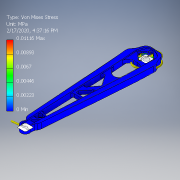
# Autodesk Inventor part: Delta_Arm
Saved by Autodesk Inventor 2019.4 (Build 234330000, 330)
## iProperties
Created: 2019-07-06
Part Number: Delta_Arm
Material: ABS Plastic
Document SubType Name: Modeling
Designer: Jorian Brusind
Density: 1.06 g/cm^3
Appearance: Chrome - Polished
Mass: 68.9986 g
Surface Area: 245.619 cm^2
Volume: 65.093 cm^3
Author: Jorian Brusind
Autodesk Inventor part; units mm, degrees
ref_plane "YZ Plane" through (0, 0, 0) normal (1, 0, 0) x (0, 1, 0)
ref_plane "XZ Plane" through (0, 0, 0) normal (0, 1, 0) x (-1, 0, 0)
ref_plane "Work Plane6" through (0, 10, 0) normal (0, 1, 0) x (1, 0, 0)
sketch "Sketch1" plane through (0, 0, 0) normal (0, 1, 0) x (-1, 0, 0)
  circle A0 centre (0, 0) radius 10
  circle A1 centre (0, -210) radius 25
  line L0 (0, -210) -> (0, 0)
  line L1 (0, 0) -> (10, 0)
  line L2 (0, 0) -> (-10, 0)
  line L3 (0, -210) -> (25, -210)
  line L4 (0, -210) -> (-25, -210)
  line L5 (25, -210) -> (10, 0)
  line L6 (-25, -210) -> (-10, 0)
  point P0 (9.9887, 0.4754)
  dimension "d0" = 20
  dimension "d2" = 50
  dimension "d50" = 210
  dimension "d51" = 210
  constraints: 14 end point, 5 point on circle, 2 centre point, 2 horizontal, 1 coincident, 1 parallel, 1 vertical
  measures "d0" diameter of A0
  measures "d2" diameter of A1
  measures "d50" distance of L0.start point (0, 0)
  measures "d51" vertical distance of L4.end L2.end
ref_plane "Work Plane5" through (0, 10, 0) normal (0, 1, 0) x (1, 0, 0)
ref_plane "Work Plane7" through (0, 10, 0) normal (0, 1, 0) x (1, 0, 0)
ref_plane "Work Plane4" through (0, 0, 0) normal (0, -1, 0) x (1, 0, 0)
ref_plane "Work Plane1" through (0, 5, 0) normal (0, -1, 0) x (1, 0, 0)
ref_plane "Work Plane3" through (0, 10, 0) normal (0, 1, 0) x (1, 0, 0)
ref_plane "Work Plane2" through (0, 0, 5) normal (0, 0, 1) x (1, 0, 0)
extrude "Extrusion8" add sketch "Sketch1" along normal blind 10 contours L1 L2 A0 | L5 A1 L0 A0 | A0 L0 L1 | L2 L0 A0 | A0 L0 A1 L6 | L5 L3 L0 A1 | A1 L0 L4 L6 | A1 L4 L3
sketch "Sketch10" plane through (0, 10, 0) normal (0, 1, 0) x (1, 0, 0)
  circle A0 centre (0, 0) radius 2
  arc A1 (25, 210) -> (-25, 210) centre (0, 210) ccw projected
  circle A2 centre (0, 210) radius 3
  dimension "d54" = 4
  dimension "d55" = 6
  constraints: 2 centre point, 2 coincident
  measures "d54" diameter of A0
  measures "d55" diameter of A2
extrude "Extrusion9" cut sketch "Sketch10" against normal blind 10
sketch "Sketch13" plane through (0, 10, 0) normal (0, 1, 0) x (1, 0, 0)
  arc A0 (-8.9826, 205.2525) -> (-4.6035, 200.9428) centre (0, 210) ccw
  arc A1 (-8.9826, 205.2525) -> (-10.7359, 206.6884) centre (-11.5651, 203.8876) ccw
  arc A2 (-10.7874, 213.1397) -> (-10.7359, 206.6884) centre (-9.7787, 209.9219) ccw
  arc A3 (-3.1397, 199.2126) -> (-4.6035, 200.9428) centre (-5.927, 198.3388) ccw
  arc A4 (-3.1397, 199.2126) -> (3.3116, 199.2641) centre (0.0781, 200.2213) ccw
  arc A5 (4.7475, 201.0174) -> (9.0572, 205.3965) centre (0, 210) ccw
  arc A6 (4.7475, 201.0174) -> (3.3116, 199.2641) centre (6.1124, 198.4349) ccw
  arc A7 (10.7874, 206.8603) -> (10.7359, 213.3116) centre (9.7787, 210.0781) ccw
  arc A8 (8.9826, 214.7475) -> (10.7359, 213.3116) centre (11.5651, 216.1124) ccw
  arc A9 (8.9826, 214.7475) -> (4.6035, 219.0572) centre (0, 210) ccw
  arc A10 (3.1397, 220.7874) -> (4.6035, 219.0572) centre (5.927, 221.6612) ccw
  arc A11 (3.1397, 220.7874) -> (-3.3116, 220.7359) centre (-0.0781, 219.7787) ccw
  arc A12 (-4.7475, 218.9826) -> (-3.3116, 220.7359) centre (-6.1124, 221.5651) ccw
  arc A13 (-4.7475, 218.9826) -> (-9.0572, 214.6035) centre (0, 210) ccw
  arc A14 (-10.7874, 213.1397) -> (-9.0572, 214.6035) centre (-11.6612, 215.927) ccw
  arc A15 (10.7874, 206.8603) -> (9.0572, 205.3965) centre (11.6612, 204.073) ccw
  arc A16 (25, 210) -> (-25, 210) centre (0, 210) ccw projected
  point P0 (0, 0)
  point P1 (-3.2721, -90.998)
  dimension "d63" = 210
  dimension "d64" = 25
  constraints: 32 point on circle, 16 centre point, 4 other
  measures "d63" distance of point (0, 0) A13.centre
  measures "d64" distance of A16.end A16.centre
extrude "Extrusion11" cut sketch "Sketch13" against normal blind 5
ref_plane "Work Plane8" through (0, 5, 0) normal (0, 1, 0) x (1, 0, 0)
sketch "Sketch15" plane through (0, 0, 0) normal (0, -1, 0) x (1, 0, 0)
  circle A0 centre (0, -210) radius 3 projected
  arc A1 (-10.7359, -206.6884) -> (-10.7874, -213.1397) centre (-9.7787, -209.9219) ccw projected
  line L0 (0, -210) -> (-9.7787, -209.9219)
  circle A2 centre (-9.7787, -209.9219) radius 1.5
  point P0 (0, 0)
  dimension "d71" = 3
  constraints: 2 end point, 1 centre point, 1 coincident
  measures "d71" diameter of A2
extrude "Extrusion13" cut sketch "Sketch15" against normal blind 10 contours A2
pattern_circular "Circular Pattern1" count 4 over 360 about axis through (0, 10, -210) along (0, -1, 0) of "Extrusion13"
sketch "Sketch16" plane through (0, 0, 0) normal (0, -1, 0) x (1, 0, 0)
  circle A0 centre (0, -210) radius 3 projected
  circle A1 centre (0, -210) radius 15
  circle A2 centre (0, 0) radius 2 projected
  circle A3 centre (0, 0) radius 5
  line L0 (0, 0) -> (-5, 0)
  line L1 (0, 0) -> (5, 0)
  line L2 (0, -210) -> (-15, -210)
  line L3 (-15, -210) -> (-5, 0)
  line L4 (0, -210) -> (15, -210)
  line L5 (15, -210) -> (5, 0)
  dimension "d77" = 30
  dimension "d78" = 10
  dimension "d79" = 15
  constraints: 12 end point, 3 horizontal, 2 coincident, 2 point on circle, 1 centre point, 1 horizontal alignment, 1 point on line, 2 other
  measures "d78" diameter of A3
  measures "d79" distance of L2.start L2.end
extrude "Extrusion14" cut sketch "Sketch16" against normal blind 2 contours L4 A1 L2 A0 | A0 L2 L3 A1 L5 L4 | L5 A1 | A1 L3 | A1 L3 A3 L5 | L1 A2 L0 A3 | A3 L0 A2 L1 | L1 L0 A2 | A2 L0 L1
mirror "Mirror3" about plane through (0, 5, 0) normal (0, 1, 0) of "Extrusion14"
sketch "Sketch17" plane through (0, 10, 0) normal (0, 1, 0) x (1, 0, 0)
  circle A0 centre (0, 0) radius 7.5
  arc A1 (-10, 0) -> (10, 0) centre (0, 0) ccw projected
  line L0 (-10, 0) -> (-10.7926, 11.0971)
  line L1 (-25, 210) -> (-10, 0) projected
  line L2 (-14.9321, 208.5747) -> (-5, 0) projected
  line L3 (10, 0) -> (25, 210) projected
  line L4 (10, 0) -> (10.9729, 13.6201)
  line L5 (-5, 11.7641) -> (-5.62, 13.0208)
  line L6 (-5.62, 13.0208) -> (-6.5713, 32.9982)
  line L7 (-6.5713, 32.9982) -> (6.4232, 29.8862)
  line L8 (5, 0) -> (14.9321, 208.5747) projected
  line L9 (6.4232, 29.8862) -> (5.7324, 15.3813)
  line L10 (5.7324, 15.3813) -> (4.634, 12.2229)
  line L11 (4.634, 12.2229) -> (-5, 11.7641)
  line L12 (-6.6817, 35.3159) -> (6.531, 32.1516)
  line L13 (-6.6817, 35.3159) -> (7.154, 45.2332)
  line L14 (-6.8056, 37.9178) -> (7.2866, 48.019)
  line L15 (6.531, 32.1516) -> (7.154, 45.2332)
  line L16 (-6.8056, 37.9178) -> (-9.1191, 86.5009)
  line L17 (7.2866, 48.019) -> (8.5353, 74.2422)
  line L18 (8.5353, 74.2422) -> (-7.9624, 62.2094)
  line L19 (8.7312, 78.3559) -> (-8.1451, 66.0469)
  line L20 (8.7312, 78.3559) -> (-9.1258, 86.6411)
  line L21 (9.0301, 84.6313) -> (-9.4009, 92.4197)
  line L22 (-9.4009, 92.4197) -> (-12.2847, 152.9795)
  line L23 (9.0301, 84.6313) -> (10.9729, 125.4301)
  line L24 (10.9729, 125.4301) -> (-12.2847, 152.9795)
  line L25 (-12.5342, 158.2184) -> (11.6288, 139.2048)
  line L26 (11.6288, 139.2048) -> (14.2227, 193.6765)
  line L27 (14.2227, 193.6765) -> (-14.1263, 191.6516)
  line L28 (-12.5342, 158.2184) -> (-14.1263, 191.6516)
  line L29 (-24.4957, 202.9397) -> (-15.4854, 210.6796)
  line L30 (-15.4854, 210.6796) -> (-15.4854, 225.5423)
  line L31 (-15.4854, 225.5423) -> (16.4712, 225.5423)
  line L32 (16.4712, 225.5423) -> (16.4712, 210)
  line L33 (16.4712, 210) -> (24.5461, 203.6459)
  line L34 (-24.4957, 202.9397) -> (-27.9273, 199.9919)
  line L35 (-27.9273, 199.9919) -> (-27.9273, 244.9368)
  line L36 (-27.9273, 244.9368) -> (27.4955, 244.9368)
  line L37 (27.4955, 244.9368) -> (27.4955, 203.6459)
  line L38 (27.4955, 203.6459) -> (24.5461, 203.6459)
  line L39 (-10.7926, 11.0971) -> (-6.0957, 7.9273)
  line L40 (10.9729, 13.6201) -> (6.8028, 7.3295)
  arc A2 (6.8028, 7.3295) -> (-6.0957, 7.9273) centre (0, 0) ccw
  arc A3 (-10, 0) -> (10, 0) centre (0, 0) ccw
  line L41 (6.8028, 7.3295) -> (5.3967, 5.2083)
  line L42 (-6.0957, 7.9273) -> (-5.2548, 5.3513)
  dimension "d83" = 15
  dimension "d84" = 20
  constraints: 79 end point, 9 point on line, 6 point on circle, 5 perpendicular, 4 parallel, 3 centre point, 2 coincident, 1 midpoint, 1 vertical, 25 other
  measures "d83" diameter of A0
  measures "d84" distance of L5.end L6.end
extrude "Extrusion15" cut sketch "Sketch17" along normal mid plane 20 contours A0 L41 L40 L3 A1 L0 L39 L42 | L2 L7 L8 L10 L11 L5 | L33 L32 L31 L30 L29 L34 L35 L36 L37 L38 | L13 L8 L12 | L2 L14 L8 L13 | L2 L18 L8 L14 | L2 L19 L8 L18 | L2 L20 L19 | L20 L2 L21 L8 | L21 L2 L24 L8 | L24 L2 L25 L8 | L25 L2 L27 L8
sketch "Sketch18" plane through (0, 2, 0) normal (0, -1, 0) x (1, 0, 0)
  line L0 (-14.9321, -208.5747) -> (-5.2548, -5.3513) projected
  line L1 (-12.2906, -153.1018) -> (10.737, -120.4763)
  line L2 (5, 0) -> (14.9321, -208.5747) projected
  line L3 (11.6438, -139.5208) -> (10.737, -120.4763)
  line L4 (9.4283, -92.9953) -> (9.2677, -89.6217)
  line L5 (9.2677, -89.6217) -> (-9.3098, -90.5063)
  line L6 (-9.3098, -90.5063) -> (8.2816, -68.9139)
  line L7 (8.2816, -68.9139) -> (8.0708, -64.4866)
  line L8 (9.4283, -92.9953) -> (-9.4712, -93.8953)
  line L9 (-9.4712, -93.8953) -> (-9.3098, -90.5063)
  line L10 (8.0708, -64.4866) -> (8.2816, -68.9139)
  line L11 (8.0708, -64.4866) -> (-9.0704, -85.4779)
  line L12 (-9.0704, -85.4779) -> (-9.3095, -90.4998)
  line L13 (10.737, -120.4763) -> (-10.737, -120.4763)
  line L14 (-10.737, -120.4763) -> (-10.5143, -115.8013)
  line L15 (-10.5143, -115.8013) -> (10.5143, -115.8013)
  line L16 (10.737, -120.4763) -> (10.5143, -115.8013)
  line L17 (11.6438, -139.5208) -> (10.737, -120.4763)
  line L18 (11.6438, -139.5208) -> (-12.7122, -161.9558)
  line L19 (-12.7122, -161.9558) -> (-12.2906, -153.1018)
  line L20 (-9.3095, -90.4998) -> (-9.0704, -85.4779)
  line L21 (-10.737, -120.4763) -> (-10.5143, -115.8013)
  line L22 (10.737, -120.4763) -> (10.5143, -115.8013)
  point P0 (0, 0)
  constraints: 42 end point, 14 point on line, 5 collinear, 2 parallel, 1 horizontal, 1 perpendicular
extrude "Extrusion16" add sketch "Sketch18" against normal blind 6 contours L0 L1 L2 L18 | L0 L5 L2 L8
sketch "Sketch19" plane through (0, 2, 0) normal (0, -1, 0) x (1, 0, 0)
  line L0 (9.4283, -92.9953) -> (-9.4712, -93.8953) projected
  line L1 (-12.2906, -153.1018) -> (10.737, -120.4763) projected
  line L2 (-9.4712, -93.8953) -> (10.737, -120.4763)
  line L3 (10.737, -120.4763) -> (6.5748, -126.3733)
  line L4 (6.5748, -126.3733) -> (-9.9808, -104.5967)
  line L5 (-5.2548, -5.3513) -> (-14.9321, -208.5747) projected
  line L6 (-9.4712, -93.8953) -> (-9.9808, -104.5967)
  line L7 (6.4232, -29.8862) -> (-5.742, -15.5817)
  line L8 (14.9321, -208.5747) -> (5, 0) projected
  line L9 (-5, -11.7641) -> (-5.62, -13.0208) projected
  line L10 (6.1866, -24.9179) -> (-5, -11.7641)
  line L11 (-5, -11.7641) -> (-5.6194, -13.007)
  line L12 (-5.7413, -15.5672) -> (-5.6194, -13.007)
  line L13 (6.1866, -24.9179) -> (6.4232, -29.8862)
  point P0 (0, 0)
  constraints: 18 end point, 2 point on line, 1 parallel, 7 other
extrude "Extrusion17" add sketch "Sketch19" against normal blind 6 contours L2 L1 L4 L5 | L7 L5 L9 L10 L8 | L9 L5 L11
fillet "Fillet4" radius 30 1 edges at (-15.4854, 5, -210.6796)
fillet "Fillet5" radius 40 1 edges at (16.4712, 5, -210)
fillet "Fillet6" radius 10 4 edges at (24.5461, 5, -203.6459) (16.4712, 5, -225.5423) (-15.4854, 5, -225.5423) (-24.4957, 5, -202.9397)
fillet "Fillet7" radius 10 4 edges at (-14.1263, 5, -191.6516) (14.2227, 5, -193.6765) (11.6438, 5, -139.5208) (-12.7122, 5, -161.9558)
fillet "Fillet8" radius 3 3 edges at (6.5748, 5, -126.3733) (-12.2906, 5, -153.1018) (-9.9808, 5, -104.5967)
fillet "Fillet9" radius 3 3 edges at (-9.4712, 5, -93.8953) (10.737, 5, -120.4763) (9.4283, 5, -92.9953)
fillet "Fillet10" radius 3 4 edges at (-9.3098, 5, -90.5063) (9.2677, 5, -89.6217) (6.531, 5, -32.1516) (-6.6817, 5, -35.3159)
fillet "Fillet11" radius 7 1 edges at (-6.0957, 5, -7.9273)
fillet "Fillet12" radius 7 1 edges at (5.3967, 5, -5.2083)
fillet "Fillet13" radius 10 2 edges at (10.9729, 5, -13.6201) (-10.7926, 5, -11.0971)
fillet "Fillet14" radius 3 3 edges at (6.4232, 5, -29.8862) (-6.5713, 5, -32.9982) (-5.742, 5, -15.5817)
fillet "Fillet15" radius 5 1 edges at (4.634, 5, -12.2229)
fillet "Fillet16" radius 1 2 edges at (6.1866, 5, -24.9179) (-5, 5, -11.7641)
body "Solid1"
